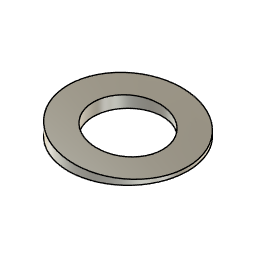
WASHER_EXT (Autodesk Fusion 360 design; units mm, degrees)
Autodesk Fusion 360 part; units mm, degrees
sketch "Esquisse1" plane through (0, 0, 0) normal (0, 0, 1) x (1, 0, 0)
  circle A0 centre (0, 0) radius 4.65
  circle A1 centre (0, 0) radius 8
  dimension "d1" = 9.3
  dimension "d2" = 16
  constraint coincident A0.centre A1.centre
  measures "d1" diameter of A0
  measures "d2" diameter of A1
extrude "Extrusion1" add sketch "Esquisse1" along normal blind 2
sketch "Esquisse2" plane through (0, 0, 0) normal (0, 1, 0) x (1, 0, 0)
  line L0 (-8.0053, -2) -> (8.0078, -0.5)
  line L1 (8.0078, -0.5) -> (8.0078, -2)
  line L2 (8.0078, -2) -> (-8.0053, -2)
  dimension "d5" = 1.5
  constraint vertical L1
  constraint perpendicular L1 L2
  measures "d5" distance of L0.end L1.end
extrude "Extrusion2" cut sketch "Esquisse2" along normal mid plane 20
